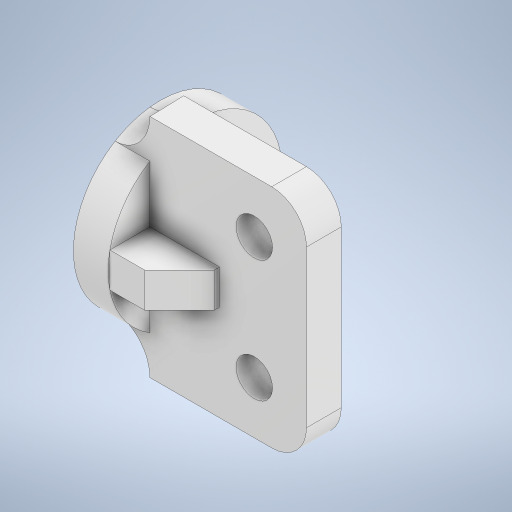
# Autodesk Inventor part: RSFF_tip_mount_1
Saved by Autodesk Inventor 2023 (Build 270158000, 158)
## iProperties
Created: 2023-06-26
Part Number: RSFF_tip_mount_1
Material: PC/ABS プラスチック
Document SubType Name: Modeling
Designer: user
Density: 0.357273 g/cm^3
Appearance: 滑らか - 白
Author: user
Autodesk Inventor part; units mm, degrees
ref_plane "YZ Plane" through (0, 0, 0) normal (1, 0, 0) x (0, 1, 0)
ref_plane "XZ Plane" through (0, 0, 0) normal (0, 1, 0) x (-1, 0, 0)
ref_plane "XY Plane" through (0, 0, 0) normal (0, 0, 1) x (1, 0, 0)
sketch "スケッチ1" plane through (0, 0, 0) normal (1, 0, 0) x (0, 1, 0)
  circle A0 centre (0, 0) radius 5
  dimension "d0" = 10
  constraints: 1 centre point, 1 coincident
  measures "d0" diameter of A0
extrude "押し出し1" add sketch "スケッチ1" along normal blind 2
sketch "スケッチ2" plane through (2, 0, 0) normal (1, 0, 0) x (0, 0, -1)
  line L0 (-2.6, 6.5) -> (-0.6, 6.5)
  line L1 (-0.6, 6.5) -> (-0.6, -6.5)
  line L2 (-0.6, -6.5) -> (-2.6, -6.5)
  line L3 (-2.6, -6.5) -> (-2.6, 6.5)
  point P0 (0, 0)
  point P1 (0.6, -6.5)
  dimension "d3" = 2
  dimension "d6" = 0.6
  dimension "d7" = 6.5
  dimension "d8" = 6.5
  constraints: 8 end point, 2 parallel, 1 horizontal, 1 perpendicular, 1 point on line
  measures "d3" distance of L0.start L0.end
  measures "d6" distance from line of point (0, 0) L1
  measures "d7" distance from line of point (0, 0) L0
  measures "d8" distance from line of point (0, 0) L2
extrude "押し出し2" add sketch "スケッチ2" along normal blind 9
sketch "スケッチ3" plane through (2, 4.2708, 2.6) normal (0, 0, 1) x (1, 0, 0)
  line L0 (0, -8.5417) -> (0, -10.7708) projected
  line L1 (0, -10.7708) -> (9, -10.7708) projected
  point P0 (-2, -4.2708)
  point P1 (6, -0.7708)
  point P2 (6, -7.7708)
  dimension "d11" = 6
  dimension "d12" = 6
  dimension "d13" = 7
  dimension "d14" = 3
  measures "d11" distance from line of L0 point (6, -0.771)
  measures "d12" distance from line of L0 point (6, -7.771)
  measures "d13" distance of point (6, -7.771) point (6, -0.771)
  measures "d14" distance from line of L1 point (6, -7.771)
hole "穴1" at (8, 3.5, 2.6) at (8, -3.5, 2.6) direction (0, 0, -1) diameter 2.1 end through all
fillet "フィレット2" radius 2 2 edges at (11, -6.5, 1.6) (11, 6.5, 1.6)
fillet "フィレット3" radius 2 2 edges at (2, 4.7244, 1.6371) (2, -4.7244, 1.6371)
sketch "スケッチ4" plane through (2, 0, 0) normal (1, 0, 0) x (0, 0, -1)
  line L0 (-2.6, -4.2708) -> (-2.6, 4.2708) projected
  arc A0 (-2.6, 4.2708) -> (-2.6, -4.2708) centre (0, 0) ccw projected
  line L1 (-2.6, 1) -> (-4.899, 1)
  line L2 (-4.899, 1) -> (-4.899, -1)
  line L3 (-4.899, -1) -> (-2.6, -1)
  line L4 (-2.6, -1) -> (-2.6, 1)
  dimension "d25" = 2
  dimension "d26" = 1
  constraints: 8 end point, 2 parallel, 1 horizontal, 1 perpendicular, 1 point on circle, 1 point on line
  measures "d25" distance of L1.end L2.end
  measures "d26" distance from line of point (0, 0) L1
extrude "押し出し3" add sketch "スケッチ4" along normal blind 4 contours L3 L2 L1 L0
chamfer "面取り1" distance 2 angle 45 1 edges at (6, 0, 4.899)
equation "\"d6\" = 0.5 * d5"
equation "\"d8\" = d7"
equation "\"d12\" = d11"
equation "\"d26\" = 0.5 * d25"
equation "\"d5\" = 1.2"
